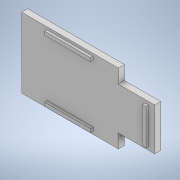
# Autodesk Inventor part: CageV5 Lid
Saved by Autodesk Inventor 2020 (Build 240168000, 168)
## iProperties
Created: 2021-03-15
Part Number: CageV5 Lid
Material: Generic
Document SubType Name: Modeling
Designer: Administrator
Density: 1 g/cm^3
Appearance: Default
Author: Administrator
Autodesk Inventor part; units mm, degrees
ref_plane "YZ Plane" through (0, 0, 0) normal (1, 0, 0) x (0, 1, 0)
ref_plane "XZ Plane" through (0, 0, 0) normal (0, 1, 0) x (-1, 0, 0)
ref_plane "XY Plane" through (0, 0, 0) normal (0, 0, 1) x (1, 0, 0)
sketch "Sketch1" plane through (0, 0, 0) normal (0, 0, 1) x (1, 0, 0)
  line L0 (-40, -29) -> (-40, 29)
  line L1 (-40, 29) -> (40, 29)
  line L2 (40, 29) -> (40, -29)
  line L3 (40, -29) -> (-40, -29)
  line L4 (-40, -29) -> (40, 29) construction
  line L5 (-40, 29) -> (40, -29) construction
  line L6 (40, 17.5) -> (70, 17.5)
  line L7 (70, 17.5) -> (70, -17.5)
  line L8 (70, -17.5) -> (40, -17.5)
  line L9 (40, -17.5) -> (40, 17.5)
  point P0 (0, 0)
  dimension "d0" = 58
  dimension "d1" = 80
  dimension "d2" = 30
  dimension "d3" = 35
  constraints: 20 end point, 4 parallel, 2 midpoint, 2 perpendicular, 1 horizontal, 1 point on line, 1 vertical
  measures "d0" distance of L0.start L0.end
  measures "d1" distance of L0.end L1.end
  measures "d2" distance of L7.end L8.end
  measures "d3" distance of L6.end L7.end
sketch "Sketch2" plane through (0, 0, 0) normal (0, 0, 1) x (1, 0, 0)
  point P0 (0, 0)
extrude "Extrusion1" add sketch "Sketch1" along normal blind 5
sketch "Sketch3" plane through (0, 0, 5) normal (0, 0, 1) x (1, 0, 0)
  line L0 (-19, 26.9) -> (19, 26.9)
  line L1 (19, 26.9) -> (19, 23.9)
  line L2 (19, 23.9) -> (-19, 23.9)
  line L3 (-19, 23.9) -> (-19, 26.9)
  line L4 (-19, -23.9) -> (19, -23.9)
  line L5 (19, -23.9) -> (19, -26.9)
  line L6 (19, -26.9) -> (-19, -26.9)
  line L7 (-19, -26.9) -> (-19, -23.9)
  line L8 (61.9, 14.9) -> (64.9, 14.9)
  line L9 (64.9, 14.9) -> (64.9, -14.9)
  line L10 (64.9, -14.9) -> (61.9, -14.9)
  line L11 (61.9, -14.9) -> (61.9, 14.9)
  line L12 (40, 29) -> (-40, 29) projected
  line L13 (-40, 29) -> (-40, -29) projected
  line L14 (40, 17.5) -> (40, 29) projected
  line L15 (-40, -29) -> (40, -29) projected
  line L16 (40, -29) -> (40, -17.5) projected
  line L17 (70, -17.5) -> (70, 17.5) projected
  line L18 (70, 17.5) -> (40, 17.5) projected
  line L19 (40, -17.5) -> (70, -17.5) projected
  point P0 (0, 0)
  dimension "d6" = 2.1
  dimension "d7" = 3
  dimension "d8" = 21
  dimension "d9" = 21
  dimension "d10" = 2.1
  dimension "d11" = 21
  dimension "d12" = 21
  dimension "d13" = 3
  dimension "d14" = 5.1
  dimension "d15" = 2.6
  dimension "d16" = 2.6
  dimension "d17" = 3
  constraints: 24 end point, 6 parallel, 3 horizontal, 3 perpendicular
  measures "d6" distance between parallel lines of L12 L0
  measures "d7" distance between parallel lines of L2 L0
  measures "d8" distance between parallel lines of L13 L3
  measures "d9" distance between parallel lines of L14 L1
  measures "d10" distance between parallel lines of L15 L6
  measures "d11" distance between parallel lines of L13 L7
  measures "d12" distance between parallel lines of L16 L5
  measures "d13" distance between parallel lines of L4 L6
  measures "d14" distance between parallel lines of L17 L9
  measures "d15" distance between parallel lines of L8 L18
  measures "d16" distance between parallel lines of L19 L10
  measures "d17" distance between parallel lines of L9 L11
extrude "Extrusion2" add sketch "Sketch3" along normal blind 2 contours L0 L1 L2 L3 | L4 L5 L6 L7 | L8 L9 L10 L11
body "Solid1"
